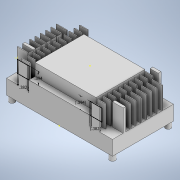
# Autodesk Inventor part: TX2 shape
Saved by Autodesk Inventor 2020 (Build 240168000, 168)
## iProperties
Created: 2019-07-20
Part Number: TX2 shape
Material: Generic
Document SubType Name: Modeling
Designer: Paul
Density: 1 g/cm^3
Appearance: Default
Author: Paul
Autodesk Inventor part; units mm, degrees
ref_plane "YZ Plane" through (0, 0, 0) normal (1, 0, 0) x (0, 1, 0)
ref_plane "XZ Plane" through (0, 0, 0) normal (0, 1, 0) x (-1, 0, 0)
ref_plane "XY Plane" through (0, 0, 0) normal (0, 0, 1) x (1, 0, 0)
sketch "Sketch1" plane through (0, 0, 0) normal (0, 1, 0) x (-1, 0, 0)
  line L0 (43.6, 25.1) -> (-43.6, 25.1)
  line L1 (-43.6, 25.1) -> (-43.6, -25.1)
  line L2 (-43.6, -25.1) -> (43.6, -25.1)
  line L3 (43.6, -25.1) -> (43.6, 25.1)
  line L4 (43.6, 25.1) -> (-43.6, -25.1) construction
  line L5 (-43.6, 25.1) -> (43.6, -25.1) construction
  point P0 (0, 0)
  dimension "d0" = 87.2
  dimension "d1" = 50.2
  constraints: 12 end point, 2 midpoint, 2 parallel, 1 horizontal, 1 perpendicular
  measures "d0" distance of L2.end L1.end
  measures "d1" distance of L1.end L0.end
extrude "Extrusion1" add sketch "Sketch1" along normal blind 30
sketch "Sketch2" plane through (0, 0, 0) normal (0, -1, 0) x (1, 0, 0)
  circle A0 centre (41.3939, 22.8369) radius 2.2
  circle A1 centre (41.3939, -22.8184) radius 2.2
  circle A2 centre (-41.2153, 22.8369) radius 2.2
  circle A3 centre (-41.2153, -22.8184) radius 2.2
  point P0 (0, 0)
  dimension "d4" = 4.4
  dimension "d5" = 4.4
  dimension "d6" = 4.4
  dimension "d7" = 4.4
  constraints: 4 centre point
  measures "d4" diameter of A0
  measures "d5" diameter of A1
  measures "d6" diameter of A2
  measures "d7" diameter of A3
extrude "Extrusion2" add sketch "Sketch2" along normal blind 4.3
sketch "Sketch3" plane through (-43.6, 0, 25.1) normal (0, 0, 1) x (1, 0, 0)
  point P0 (43.6, 0)
sketch "Sketch4" plane through (0, 30, 0) normal (0, 1, 0) x (1, 0, 0)
  line L0 (43.6, 25.1) -> (-43.6, 25.1) projected
  line L1 (43.6, 25.1) -> (34.8, 25.1)
  line L2 (34.8, 25.1) -> (34.8, 16.3)
  line L3 (34.8, 16.3) -> (43.6, 16.3)
  line L4 (43.6, 16.3) -> (43.6, 25.1)
  line L5 (-43.6, 25.1) -> (-34.8, 25.1)
  line L6 (-34.8, 25.1) -> (-34.8, 16.3)
  line L7 (-34.8, 16.3) -> (-43.6, 16.3)
  line L8 (-43.6, 16.3) -> (-43.6, 25.1)
  point P0 (0, 0)
  dimension "d10" = 8.8
  dimension "d11" = 8.8
  dimension "d14" = 8.8
  dimension "d15" = 8.8
  constraints: 16 end point, 4 parallel, 2 horizontal, 2 perpendicular
  measures "d10" distance of L3.end L2.end
  measures "d11" distance of L2.end L1.end
  measures "d14" distance of L6.end L7.end
  measures "d15" distance of L5.end L6.end
sketch "Sketch5" plane through (0, 30, 0) normal (0, 1, 0) x (1, 0, 0)
  line L0 (-43.6, -25.1) -> (43.6, -25.1) projected
  line L1 (43.6, -25.1) -> (34.8, -25.1)
  line L2 (34.8, -25.1) -> (34.8, -16.3)
  line L3 (34.8, -16.3) -> (43.6, -16.3)
  line L4 (43.6, -16.3) -> (43.6, -25.1)
  line L5 (-43.6, 25.1) -> (-43.6, -25.1) projected
  line L6 (-43.6, -25.1) -> (-34.8, -25.1)
  line L7 (-34.8, -25.1) -> (-34.8, -16.3)
  line L8 (-34.8, -16.3) -> (-43.6, -16.3)
  line L9 (-43.6, -16.3) -> (-43.6, -25.1)
  point P0 (0, 0)
  dimension "d18" = 8.8
  dimension "d19" = 8.8
  dimension "d20" = 8.8
  dimension "d21" = 8.8
  constraints: 16 end point, 4 parallel, 2 horizontal, 2 perpendicular
  measures "d18" distance of L2.end L3.end
  measures "d19" distance of L1.end L2.end
  measures "d20" distance of L8.end L7.end
  measures "d21" distance of L7.end L6.end
extrude "Extrusion3" cut sketch "Sketch4" against normal blind 18
extrude "Extrusion4" cut sketch "Sketch5" against normal blind 18
sketch "Sketch6" plane through (43.6, 0, -25.1) normal (0, 0, -1) x (-1, 0, 0)
  line L0 (78.4, 30) -> (8.8, 30) projected
  line L1 (8.8, 30) -> (18.5, 30)
  line L2 (18.5, 30) -> (18.5, 20)
  line L3 (18.5, 20) -> (8.8, 20)
  line L4 (8.8, 20) -> (8.8, 30)
  line L5 (78.4, 30) -> (68.7, 30)
  line L6 (68.7, 30) -> (68.7, 20)
  line L7 (68.7, 20) -> (78.4, 20)
  line L8 (78.4, 20) -> (78.4, 30)
  line L9 (18.5, 30) -> (68.7, 30)
  line L10 (68.7, 30) -> (68.7, 20)
  line L11 (68.7, 20) -> (18.5, 20)
  line L12 (18.5, 20) -> (18.5, 30)
  point P0 (43.6, 0)
  point P1 (18.5, 20)
  point P2 (18.5, 30)
  dimension "d26" = 9.7
  dimension "d27" = 10
  dimension "d28" = 9.7
  dimension "d29" = 10
  constraints: 24 end point, 6 parallel, 3 horizontal, 3 perpendicular
  measures "d26" distance of L2.end L3.end
  measures "d27" distance of L1.end L2.end
  measures "d28" distance of L7.end L6.end
  measures "d29" distance of L6.end L5.end
extrude "Extrusion5" cut sketch "Sketch6" against normal blind 5 contours L6 L11 L2 L0
sketch "Sketch7" plane through (-43.6, 0, 25.1) normal (0, 0, 1) x (1, 0, 0)
  line L0 (0, 30) -> (8.8, 30) projected
  line L1 (8.8, 30) -> (18.5, 30)
  line L2 (18.5, 30) -> (18.5, 20)
  line L3 (18.5, 20) -> (8.8, 20)
  line L4 (8.8, 20) -> (8.8, 30)
  line L5 (78.4, 12) -> (78.4, 30) projected
  line L6 (78.4, 30) -> (68.7, 30)
  line L7 (68.7, 30) -> (68.7, 20)
  line L8 (68.7, 20) -> (78.4, 20)
  line L9 (78.4, 20) -> (78.4, 30)
  line L10 (18.5, 30) -> (68.7, 30)
  line L11 (68.7, 30) -> (68.7, 20)
  line L12 (68.7, 20) -> (18.5, 20)
  line L13 (18.5, 20) -> (18.5, 30)
  point P0 (43.6, 0)
  point P1 (18.5, 20)
  dimension "d32" = 9.7
  dimension "d33" = 10
  dimension "d34" = 9.7
  dimension "d35" = 10
  constraints: 24 end point, 6 parallel, 3 horizontal, 3 perpendicular
  measures "d32" distance of L2.end L3.end
  measures "d33" distance of L1.end L2.end
  measures "d34" distance of L8.end L7.end
  measures "d35" distance of L7.end L6.end
extrude "Extrusion6" cut sketch "Sketch7" along normal blind 5 contours L10 L7 L12 L2
sketch "Sketch8" plane through (-43.6, 0, 25.1) normal (0, 0, 1) x (1, 0, 0)
  point P0 (43.6, 0)
sketch "Sketch9" plane through (-43.6, 0, 25.1) normal (0, 0, 1) x (1, 0, 0)
  line L0 (8.8, 30) -> (18.5, 30)
  line L1 (18.5, 30) -> (18.5, 20)
  line L2 (18.5, 20) -> (8.8, 20)
  line L3 (8.8, 20) -> (8.8, 30)
  line L4 (78.4, 30) -> (68.7, 30) projected
  line L5 (68.7, 20) -> (68.7, 30) projected
  line L6 (78.4, 30) -> (68.7, 30)
  line L7 (68.7, 30) -> (68.7, 20)
  line L8 (68.7, 20) -> (78.4, 20)
  line L9 (78.4, 20) -> (78.4, 30)
  point P0 (43.6, 0)
  dimension "d38" = 9.7
  dimension "d39" = 10
  dimension "d40" = 9.7
  dimension "d41" = 10
  constraints: 16 end point, 4 parallel, 2 horizontal, 2 perpendicular
  measures "d38" distance of L1.end L2.end
  measures "d39" distance of L0.end L1.end
  measures "d40" distance of L8.end L5.start
  measures "d41" distance of L5.start L6.end
sketch "Sketch10" plane through (-43.6, 0, 25.1) normal (0, 0, 1) x (1, 0, 0)
  line L0 (68.7, 30) -> (18.5, 30) projected
  line L1 (18.5, 20) -> (68.7, 20) projected
  line L2 (18.5, 30) -> (68.7, 30)
  line L3 (68.7, 30) -> (68.7, 20)
  line L4 (68.7, 20) -> (18.5, 20)
  line L5 (18.5, 20) -> (18.5, 30)
  point P0 (43.6, 0)
  constraints: 8 end point, 2 parallel, 1 horizontal, 1 perpendicular
extrude "Extrusion7" cut sketch "Sketch10" against normal blind 5
sketch "Sketch11" plane through (0, 30, 0) normal (0, 1, 0) x (1, 0, 0)
  line L0 (25.1, -25.1) -> (-25.1, -25.1) projected
  line L1 (25.1, -25.1) -> (26.6, -25.1)
  line L2 (26.6, -25.1) -> (26.6, 25.1)
  line L3 (26.6, 25.1) -> (25.1, 25.1)
  line L4 (25.1, 25.1) -> (25.1, -25.1)
  line L5 (-25.1, -25.1) -> (-26.6, -25.1)
  line L6 (-26.6, -25.1) -> (-26.6, 25.1)
  line L7 (-26.6, 25.1) -> (-25.1, 25.1)
  line L8 (-25.1, 25.1) -> (-25.1, -25.1)
  point P0 (0, 0)
  dimension "d44" = 1.5
  dimension "d45" = 50.2
  dimension "d46" = 1.5
  constraints: 16 end point, 4 parallel, 2 horizontal, 2 perpendicular
  measures "d44" distance of L3.end L2.end
  measures "d45" distance of L2.end L1.end
  measures "d46" distance of L6.end L7.end
extrude "Extrusion8" cut sketch "Sketch11" against normal blind 18
sketch "Sketch12" plane through (0, 30, 0) normal (0, 1, 0) x (1, 0, 0)
  line L0 (-34.8, 25.1) -> (-33.3, 25.1)
  line L1 (-33.3, 25.1) -> (-33.3, -25.1)
  line L2 (-33.3, -25.1) -> (-34.8, -25.1)
  line L3 (-34.8, -25.1) -> (-34.8, 25.1)
  line L4 (34.8, 25.1) -> (43.6, 25.1) projected
  line L5 (34.8, 25.1) -> (33.3, 25.1)
  line L6 (33.3, 25.1) -> (33.3, -25.1)
  line L7 (33.3, -25.1) -> (34.8, -25.1)
  line L8 (34.8, -25.1) -> (34.8, 25.1)
  point P0 (0, 0)
  dimension "d50" = 1.5
  dimension "d51" = 50.2
  dimension "d52" = 1.5
  dimension "d53" = 50.2
  constraints: 16 end point, 4 parallel, 2 horizontal, 2 perpendicular
  measures "d50" distance of L1.end L2.end
  measures "d51" distance of L0.end L1.end
  measures "d52" distance of L7.end L6.end
  measures "d53" distance of L6.end L5.end
extrude "Extrusion9" cut sketch "Sketch12" against normal blind 18
sketch "Sketch13" plane through (0, 30, 0) normal (0, 1, 0) x (1, 0, 0)
  line L0 (-34.8, -16.3) -> (-34.8, 16.3) projected
  line L1 (-43.6, 16.3) -> (-43.6, -16.3) projected
  line L2 (-43.6, 16.3) -> (-34.81, 16.3)
  line L3 (-34.81, 16.3) -> (-34.81, 15.65)
  line L4 (-34.81, 15.65) -> (-43.6, 15.65)
  line L5 (-43.6, 15.65) -> (-43.6, 16.3)
  line L6 (-43.6, 15.65) -> (179.412, 15.65)
  line L7 (179.412, 15.65) -> (179.412, 11.95)
  line L8 (179.412, 11.95) -> (-43.6, 11.95)
  line L9 (-43.6, 11.95) -> (-43.6, 15.65)
  line L10 (-43.6, 11.95) -> (-34.81, 11.95)
  line L11 (-34.81, 11.95) -> (-34.81, 11.3)
  line L12 (-34.81, 11.3) -> (-43.6, 11.3)
  line L13 (-43.6, 11.3) -> (-43.6, 11.95)
  line L14 (-43.6, 11.3) -> (-34.81, 11.3)
  line L15 (-34.81, 11.3) -> (-34.81, 7.6)
  line L16 (-34.81, 7.6) -> (-43.6, 7.6)
  line L17 (-43.6, 7.6) -> (-43.6, 11.3)
  line L18 (-43.6, 7.6) -> (-34.81, 7.6)
  line L19 (-34.81, 7.6) -> (-34.81, 6.95)
  line L20 (-34.81, 6.95) -> (-43.6, 6.95)
  line L21 (-43.6, 6.95) -> (-43.6, 7.6)
  line L22 (-43.6, 6.95) -> (-34.81, 6.95)
  line L23 (-34.81, 6.95) -> (-34.81, 3.25)
  line L24 (-34.81, 3.25) -> (-43.6, 3.25)
  line L25 (-43.6, 3.25) -> (-43.6, 6.95)
  line L26 (-43.6, 3.25) -> (-34.81, 3.25)
  line L27 (-34.81, 3.25) -> (-34.81, 2.6)
  line L28 (-34.81, 2.6) -> (-43.6, 2.6)
  line L29 (-43.6, 2.6) -> (-43.6, 3.25)
  line L30 (-43.6, 2.6) -> (-34.81, 2.6)
  line L31 (-34.81, 2.6) -> (-34.81, -1.1)
  line L32 (-34.81, -1.1) -> (-43.6, -1.1)
  line L33 (-43.6, -1.1) -> (-43.6, 2.6)
  line L34 (-43.6, -1.1) -> (-34.81, -1.1)
  line L35 (-34.81, -1.1) -> (-34.81, -1.75)
  line L36 (-34.81, -1.75) -> (-43.6, -1.75)
  line L37 (-43.6, -1.75) -> (-43.6, -1.1)
  line L38 (-43.6, -1.75) -> (-34.81, -1.75)
  line L39 (-34.81, -1.75) -> (-34.81, -5.45)
  line L40 (-34.81, -5.45) -> (-43.6, -5.45)
  line L41 (-43.6, -5.45) -> (-43.6, -1.75)
  line L42 (-43.6, -5.45) -> (-34.81, -5.45)
  line L43 (-34.81, -5.45) -> (-34.81, -6.1)
  line L44 (-34.81, -6.1) -> (-43.6, -6.1)
  line L45 (-43.6, -6.1) -> (-43.6, -5.45)
  line L46 (-43.6, -6.1) -> (-34.81, -6.1)
  line L47 (-34.81, -6.1) -> (-34.81, -9.8)
  line L48 (-34.81, -9.8) -> (-43.6, -9.8)
  line L49 (-43.6, -9.8) -> (-43.6, -6.1)
  line L50 (-43.6, -9.8) -> (-34.81, -9.8)
  line L51 (-34.81, -9.8) -> (-34.81, -10.45)
  line L52 (-34.81, -10.45) -> (-43.6, -10.45)
  line L53 (-43.6, -10.45) -> (-43.6, -9.8)
  line L54 (-43.6, -16.3) -> (-34.8, -16.3) projected
  line L55 (-43.6, -16.3) -> (-34.81, -16.3)
  line L56 (-34.81, -16.3) -> (-34.81, -15.65)
  line L57 (-34.81, -15.65) -> (-43.6, -15.65)
  line L58 (-43.6, -15.65) -> (-43.6, -16.3)
  line L59 (-43.6, -15.65) -> (-34.81, -15.65)
  line L60 (-34.81, -15.65) -> (-34.81, -11.95)
  line L61 (-34.81, -11.95) -> (-43.6, -11.95)
  line L62 (-43.6, -11.95) -> (-43.6, -15.65)
  point P0 (0, 0)
  point P1 (-34.8, 11.95)
  point P2 (-34.8, 15.65)
  point P3 (-43.6, 11.95)
  dimension "d56" = 8.8
  dimension "d57" = 8.79
  dimension "d58" = 0.65
  dimension "d59" = 223.012
  dimension "d60" = 3.7
  dimension "d61" = 8.79
  dimension "d62" = 0.65
  dimension "d63" = 8.79
  dimension "d64" = 3.7
  dimension "d65" = 8.79
  dimension "d66" = 0.65
  dimension "d67" = 8.79
  dimension "d68" = 3.7
  dimension "d69" = 8.79
  dimension "d70" = 0.65
  dimension "d71" = 8.79
  dimension "d72" = 3.7
  dimension "d73" = 8.79
  dimension "d74" = 0.65
  dimension "d75" = 8.79
  dimension "d76" = 3.7
  dimension "d77" = 8.79
  dimension "d78" = 0.65
  dimension "d79" = 8.79
  dimension "d80" = 3.7
  dimension "d81" = 8.79
  dimension "d82" = 0.65
  dimension "d83" = 8.79
  dimension "d84" = 0.65
  dimension "d85" = 8.79
  dimension "d86" = 3.7
  constraints: 120 end point, 30 parallel, 15 horizontal, 15 perpendicular
  measures "d56" distance between parallel lines of L0 L1
  measures "d57" distance of L3.end L4.end
  measures "d58" distance of L2.end L3.end
  measures "d59" distance of L7.end L8.end
  measures "d60" distance of L6.end L7.end
  measures "d61" distance of L11.end L12.end
  measures "d62" distance of L10.end L11.end
  measures "d63" distance of L15.end L16.end
  measures "d64" distance of L14.end L15.end
  measures "d65" distance of L19.end L20.end
  measures "d66" distance of L18.end L19.end
  measures "d67" distance of L23.end L24.end
  measures "d68" distance of L22.end L23.end
  measures "d69" distance of L27.end L28.end
  measures "d70" distance of L26.end L27.end
  measures "d71" distance of L31.end L32.end
  measures "d72" distance of L30.end L31.end
  measures "d73" distance of L35.end L36.end
  measures "d74" distance of L34.end L35.end
  measures "d75" distance of L39.end L40.end
  measures "d76" distance of L38.end L39.end
  measures "d77" distance of L43.end L44.end
  measures "d78" distance of L42.end L43.end
  measures "d79" distance of L47.end L48.end
  measures "d80" distance of L46.end L47.end
  measures "d81" distance of L51.end L52.end
  measures "d82" distance of L50.end L51.end
  measures "d83" distance of L57.end L56.end
  measures "d84" distance of L56.end L55.end
  measures "d85" distance of L61.end L60.end
  measures "d86" distance of L60.end L59.end
extrude "Extrusion10" cut sketch "Sketch13" against normal blind 18 contours L8 L1 L4 L6 L0 | L57 L1 L61 L60 | L15 L16 L1 L12 | L23 L24 L1 L20 | L1 L44 L47 L48 | L31 L32 L1 L28 | L1 L36 L39 L40
sketch "Sketch14" plane through (0, 30, 0) normal (0, 1, 0) x (1, 0, 0)
  line L0 (43.6, 16.3) -> (34.8, 16.3) projected
  line L1 (34.8, 16.3) -> (43.6, 16.3)
  line L2 (43.6, 16.3) -> (43.6, 15.65)
  line L3 (43.6, 15.65) -> (34.8, 15.65)
  line L4 (34.8, 15.65) -> (34.8, 16.3)
  line L5 (34.8, 15.65) -> (43.6, 15.65)
  line L6 (43.6, 15.65) -> (43.6, 11.95)
  line L7 (43.6, 11.95) -> (34.8, 11.95)
  line L8 (34.8, 11.95) -> (34.8, 15.65)
  line L9 (34.8, 11.95) -> (43.6, 11.95)
  line L10 (43.6, 11.95) -> (43.6, 11.3)
  line L11 (43.6, 11.3) -> (34.8, 11.3)
  line L12 (34.8, 11.3) -> (34.8, 11.95)
  point P0 (0, 0)
  dimension "d89" = 8.8
  dimension "d90" = 0.65
  dimension "d91" = 8.8
  dimension "d92" = 3.7
  dimension "d93" = 8.8
  dimension "d94" = 0.65
  constraints: 24 end point, 6 parallel, 3 horizontal, 3 perpendicular
  measures "d89" distance of L2.end L3.end
  measures "d90" distance of L1.end L2.end
  measures "d91" distance of L6.end L7.end
  measures "d92" distance of L5.end L6.end
  measures "d93" distance of L10.end L11.end
  measures "d94" distance of L9.end L10.end
extrude "Extrusion11" cut sketch "Sketch14" against normal blind 18 contours L6 L7 L8 L3
sketch "Sketch15" plane through (0, 30, 0) normal (0, 1, 0) x (1, 0, 0)
  line L0 (43.6, 11.95) -> (34.8, 11.95) projected
  line L1 (34.8, 11.95) -> (43.6, 11.95)
  line L2 (43.6, 11.95) -> (43.6, 11.3)
  line L3 (43.6, 11.3) -> (34.8, 11.3)
  line L4 (34.8, 11.3) -> (34.8, 11.95)
  line L5 (34.8, 11.3) -> (43.6, 11.3)
  line L6 (43.6, 11.3) -> (43.6, 7.6)
  line L7 (43.6, 7.6) -> (34.8, 7.6)
  line L8 (34.8, 7.6) -> (34.8, 11.3)
  line L9 (34.8, 7.6) -> (43.6, 7.6)
  line L10 (43.6, 7.6) -> (43.6, 6.95)
  line L11 (43.6, 6.95) -> (34.8, 6.95)
  line L12 (34.8, 6.95) -> (34.8, 7.6)
  line L13 (34.8, 6.95) -> (43.6, 6.95)
  line L14 (43.6, 6.95) -> (43.6, 3.25)
  line L15 (43.6, 3.25) -> (34.8, 3.25)
  line L16 (34.8, 3.25) -> (34.8, 6.95)
  line L17 (34.8, 3.25) -> (43.6, 3.25)
  line L18 (43.6, 3.25) -> (43.6, 2.6)
  line L19 (43.6, 2.6) -> (34.8, 2.6)
  line L20 (34.8, 2.6) -> (34.8, 3.25)
  line L21 (34.8, 2.6) -> (43.6, 2.6)
  line L22 (43.6, 2.6) -> (43.6, -1.1)
  line L23 (43.6, -1.1) -> (34.8, -1.1)
  line L24 (34.8, -1.1) -> (34.8, 2.6)
  line L25 (34.8, -1.1) -> (43.6, -1.1)
  line L26 (43.6, -1.1) -> (43.6, -1.75)
  line L27 (43.6, -1.75) -> (34.8, -1.75)
  line L28 (34.8, -1.75) -> (34.8, -1.1)
  line L29 (34.8, -1.75) -> (43.6, -1.75)
  line L30 (43.6, -1.75) -> (43.6, -5.45)
  line L31 (43.6, -5.45) -> (34.8, -5.45)
  line L32 (34.8, -5.45) -> (34.8, -1.75)
  line L33 (34.8, -5.45) -> (43.6, -5.45)
  line L34 (43.6, -5.45) -> (43.6, -6.1)
  line L35 (43.6, -6.1) -> (34.8, -6.1)
  line L36 (34.8, -6.1) -> (34.8, -5.45)
  line L37 (34.8, -6.1) -> (43.6, -6.1)
  line L38 (43.6, -6.1) -> (43.6, -9.8)
  line L39 (43.6, -9.8) -> (34.8, -9.8)
  line L40 (34.8, -9.8) -> (34.8, -6.1)
  line L41 (34.8, -9.8) -> (43.6, -9.8)
  line L42 (43.6, -9.8) -> (43.6, -10.45)
  line L43 (43.6, -10.45) -> (34.8, -10.45)
  line L44 (34.8, -10.45) -> (34.8, -9.8)
  line L45 (34.8, 11.95) -> (34.8, -16.3) projected
  line L46 (34.8, -16.3) -> (43.6, -16.3)
  line L47 (43.6, -16.3) -> (43.6, -15.65)
  line L48 (43.6, -15.65) -> (34.8, -15.65)
  line L49 (34.8, -15.65) -> (34.8, -16.3)
  line L50 (34.8, -10.45) -> (43.6, -10.45)
  line L51 (43.6, -10.45) -> (43.6, -14.15)
  line L52 (43.6, -14.15) -> (34.8, -14.15)
  line L53 (34.8, -14.15) -> (34.8, -10.45)
  point P0 (0, 0)
  dimension "d97" = 8.8
  dimension "d98" = 0.65
  dimension "d99" = 8.8
  dimension "d100" = 3.7
  dimension "d101" = 8.8
  dimension "d102" = 0.65
  dimension "d103" = 8.8
  dimension "d104" = 3.7
  dimension "d105" = 8.8
  dimension "d106" = 0.65
  dimension "d107" = 8.8
  dimension "d108" = 3.7
  dimension "d109" = 8.8
  dimension "d110" = 0.65
  dimension "d111" = 8.8
  dimension "d112" = 3.7
  dimension "d113" = 8.8
  dimension "d114" = 0.65
  dimension "d115" = 8.8
  dimension "d116" = 3.7
  dimension "d117" = 8.8
  dimension "d118" = 0.65
  dimension "d119" = 8.8
  dimension "d120" = 0.65
  dimension "d121" = 8.8
  dimension "d122" = 3.7
  constraints: 104 end point, 26 parallel, 13 horizontal, 13 perpendicular, 1 other
  measures "d97" distance of L2.end L3.end
  measures "d98" distance of L1.end L2.end
  measures "d99" distance of L6.end L7.end
  measures "d100" distance of L5.end L6.end
  measures "d101" distance of L10.end L11.end
  measures "d102" distance of L9.end L10.end
  measures "d103" distance of L14.end L15.end
  measures "d104" distance of L13.end L14.end
  measures "d105" distance of L18.end L19.end
  measures "d106" distance of L17.end L18.end
  measures "d107" distance of L22.end L23.end
  measures "d108" distance of L21.end L22.end
  measures "d109" distance of L26.end L27.end
  measures "d110" distance of L25.end L26.end
  measures "d111" distance of L30.end L31.end
  measures "d112" distance of L29.end L30.end
  measures "d113" distance of L34.end L35.end
  measures "d114" distance of L33.end L34.end
  measures "d115" distance of L38.end L39.end
  measures "d116" distance of L37.end L38.end
  measures "d117" distance of L42.end L43.end
  measures "d118" distance of L41.end L42.end
  measures "d119" distance of L48.end L47.end
  measures "d120" distance of L47.end L46.end
  measures "d121" distance of L51.end L52.end
  measures "d122" distance of L50.end L51.end
extrude "Extrusion12" cut sketch "Sketch15" against normal blind 18 contours L6 L7 L8 L3 | L14 L15 L16 L11 | L22 L23 L24 L19 | L30 L31 L32 L27 | L38 L39 L40 L35 | L51 L52 L45 L43
sketch "Sketch16" plane through (0, 30, 0) normal (0, 1, 0) x (1, 0, 0)
  line L0 (-33.3, 25.1) -> (-33.3, -25.1) projected
  line L1 (-26.6, -25.1) -> (-26.6, 25.1) projected
  line L2 (-33.3, 25.1) -> (-26.59, 25.1)
  line L3 (-26.59, 25.1) -> (-26.59, 24.45)
  line L4 (-26.59, 24.45) -> (-33.3, 24.45)
  line L5 (-33.3, 24.45) -> (-33.3, 25.1)
  line L6 (-33.3, 24.45) -> (-26.59, 24.45)
  line L7 (-26.59, 24.45) -> (-26.59, 20.75)
  line L8 (-26.59, 20.75) -> (-33.3, 20.75)
  line L9 (-33.3, 20.75) -> (-33.3, 24.45)
  line L10 (-33.3, 20.75) -> (-26.59, 20.75)
  line L11 (-26.59, 20.75) -> (-26.59, 20.1)
  line L12 (-26.59, 20.1) -> (-33.3, 20.1)
  line L13 (-33.3, 20.1) -> (-33.3, 20.75)
  point P0 (0, 0)
  point P1 (-26.6, 20.75)
  point P2 (-26.6, 24.45)
  dimension "d125" = 6.71
  dimension "d126" = 0.65
  dimension "d127" = 6.71
  dimension "d128" = 3.7
  dimension "d129" = 6.71
  dimension "d130" = 0.65
  constraints: 24 end point, 6 parallel, 3 horizontal, 3 perpendicular
  measures "d125" distance of L3.end L4.end
  measures "d126" distance of L2.end L3.end
  measures "d127" distance of L7.end L8.end
  measures "d128" distance of L6.end L7.end
  measures "d129" distance of L11.end L12.end
  measures "d130" distance of L10.end L11.end
extrude "Extrusion13" cut sketch "Sketch16" against normal blind 18 contours L4 L1 L8 L0
sketch "Sketch17" plane through (0, 30, 0) normal (0, 1, 0) x (1, 0, 0)
  line L0 (-26.6, 20.75) -> (-33.3, 20.75) projected
  line L1 (-33.3, 20.75) -> (-26.59, 20.75)
  line L2 (-26.59, 20.75) -> (-26.59, 20.1)
  line L3 (-26.59, 20.1) -> (-33.3, 20.1)
  line L4 (-33.3, 20.1) -> (-33.3, 20.75)
  line L5 (-33.3, 20.1) -> (-26.59, 20.1)
  line L6 (-26.59, 20.1) -> (-26.59, 16.4)
  line L7 (-26.59, 16.4) -> (-33.3, 16.4)
  line L8 (-33.3, 16.4) -> (-33.3, 20.1)
  line L9 (-33.3, 16.4) -> (-26.59, 16.4)
  line L10 (-26.59, 16.4) -> (-26.59, 15.75)
  line L11 (-26.59, 15.75) -> (-33.3, 15.75)
  line L12 (-33.3, 15.75) -> (-33.3, 16.4)
  line L13 (-33.3, 15.75) -> (-26.59, 15.75)
  line L14 (-26.59, 15.75) -> (-26.59, 12.05)
  line L15 (-26.59, 12.05) -> (-33.3, 12.05)
  line L16 (-33.3, 12.05) -> (-33.3, 15.75)
  line L17 (-33.3, 12.05) -> (-26.59, 12.05)
  line L18 (-26.59, 12.05) -> (-26.59, 11.4)
  line L19 (-26.59, 11.4) -> (-33.3, 11.4)
  line L20 (-33.3, 11.4) -> (-33.3, 12.05)
  line L21 (-33.3, 11.4) -> (-26.59, 11.4)
  line L22 (-26.59, 11.4) -> (-26.59, 7.7)
  line L23 (-26.59, 7.7) -> (-33.3, 7.7)
  line L24 (-33.3, 7.7) -> (-33.3, 11.4)
  line L25 (-33.3, 7.7) -> (-26.59, 7.7)
  line L26 (-26.59, 7.7) -> (-26.59, 7.05)
  line L27 (-26.59, 7.05) -> (-33.3, 7.05)
  line L28 (-33.3, 7.05) -> (-33.3, 7.7)
  line L29 (-33.3, 7.05) -> (-26.59, 7.05)
  line L30 (-26.59, 7.05) -> (-26.59, 3.35)
  line L31 (-26.59, 3.35) -> (-33.3, 3.35)
  line L32 (-33.3, 3.35) -> (-33.3, 7.05)
  line L33 (-33.3, 3.35) -> (-26.59, 3.35)
  line L34 (-26.59, 3.35) -> (-26.59, 2.7)
  line L35 (-26.59, 2.7) -> (-33.3, 2.7)
  line L36 (-33.3, 2.7) -> (-33.3, 3.35)
  line L37 (-33.3, 2.7) -> (-26.59, 2.7)
  line L38 (-26.59, 2.7) -> (-26.59, -1)
  line L39 (-26.59, -1) -> (-33.3, -1)
  line L40 (-33.3, -1) -> (-33.3, 2.7)
  line L41 (-33.3, -1) -> (-26.59, -1)
  line L42 (-26.59, -1) -> (-26.59, -1.65)
  line L43 (-26.59, -1.65) -> (-33.3, -1.65)
  line L44 (-33.3, -1.65) -> (-33.3, -1)
  line L45 (-33.3, -1.65) -> (-26.59, -1.65)
  line L46 (-26.59, -1.65) -> (-26.59, -5.35)
  line L47 (-26.59, -5.35) -> (-33.3, -5.35)
  line L48 (-33.3, -5.35) -> (-33.3, -1.65)
  line L49 (-33.3, -5.35) -> (-26.59, -5.35)
  line L50 (-26.59, -5.35) -> (-26.59, -6)
  line L51 (-26.59, -6) -> (-33.3, -6)
  line L52 (-33.3, -6) -> (-33.3, -5.35)
  line L53 (-33.3, -6) -> (-26.59, -6)
  line L54 (-26.59, -6) -> (-26.59, -9.7)
  line L55 (-26.59, -9.7) -> (-33.3, -9.7)
  line L56 (-33.3, -9.7) -> (-33.3, -6)
  line L57 (-33.3, -9.7) -> (-26.59, -9.7)
  line L58 (-26.59, -9.7) -> (-26.59, -10.35)
  line L59 (-26.59, -10.35) -> (-33.3, -10.35)
  line L60 (-33.3, -10.35) -> (-33.3, -9.7)
  line L61 (-33.3, -10.35) -> (-26.59, -10.35)
  line L62 (-26.59, -10.35) -> (-26.59, -13.4782)
  line L63 (-26.59, -13.4782) -> (-33.3, -13.4782)
  line L64 (-33.3, -13.4782) -> (-33.3, -10.35)
  line L65 (-33.3, -13.4782) -> (-26.59, -13.4782)
  line L66 (-26.59, -13.4782) -> (-26.59, -14.1282)
  line L67 (-26.59, -14.1282) -> (-33.3, -14.1282)
  line L68 (-33.3, -14.1282) -> (-33.3, -13.4782)
  line L69 (-33.3, -14.1282) -> (-26.59, -14.1282)
  line L70 (-26.59, -14.1282) -> (-26.59, -17.8282)
  line L71 (-26.59, -17.8282) -> (-33.3, -17.8282)
  line L72 (-33.3, -17.8282) -> (-33.3, -14.1282)
  line L73 (-33.3, -17.8282) -> (-26.59, -17.8282)
  line L74 (-26.59, -17.8282) -> (-26.59, -18.4782)
  line L75 (-26.59, -18.4782) -> (-33.3, -18.4782)
  line L76 (-33.3, -18.4782) -> (-33.3, -17.8282)
  line L77 (-33.3, -18.4782) -> (-26.59, -18.4782)
  line L78 (-26.59, -18.4782) -> (-26.59, -22.1782)
  line L79 (-26.59, -22.1782) -> (-33.3, -22.1782)
  line L80 (-33.3, -22.1782) -> (-33.3, -18.4782)
  line L81 (-33.3, -22.1782) -> (-26.59, -22.1782)
  line L82 (-26.59, -22.1782) -> (-26.59, -22.8282)
  line L83 (-26.59, -22.8282) -> (-33.3, -22.8282)
  line L84 (-33.3, -22.8282) -> (-33.3, -22.1782)
  line L85 (-33.3, 20.75) -> (-33.3, -25.1) projected
  line L86 (-33.3, -25.1) -> (-26.59, -25.1)
  line L87 (-26.59, -25.1) -> (-26.59, -24.45)
  line L88 (-26.59, -24.45) -> (-33.3, -24.45)
  line L89 (-33.3, -24.45) -> (-33.3, -25.1)
  point P0 (0, 0)
  dimension "d133" = 6.71
  dimension "d134" = 0.65
  dimension "d135" = 6.71
  dimension "d136" = 3.7
  dimension "d137" = 6.71
  dimension "d138" = 0.65
  dimension "d139" = 6.71
  dimension "d140" = 3.7
  dimension "d141" = 6.71
  dimension "d142" = 0.65
  dimension "d143" = 6.71
  dimension "d144" = 3.7
  dimension "d145" = 6.71
  dimension "d146" = 0.65
  dimension "d147" = 6.71
  dimension "d148" = 3.7
  dimension "d149" = 6.71
  dimension "d150" = 0.65
  dimension "d151" = 6.71
  dimension "d152" = 3.7
  dimension "d153" = 6.71
  dimension "d154" = 0.65
  dimension "d155" = 6.71
  dimension "d156" = 3.7
  dimension "d157" = 6.71
  dimension "d158" = 0.65
  dimension "d159" = 6.71
  dimension "d160" = 3.7
  dimension "d161" = 6.71
  dimension "d162" = 0.65
  dimension "d163" = 6.71
  dimension "d164" = 6.71
  dimension "d165" = 0.65
  dimension "d166" = 6.71
  dimension "d167" = 3.7
  dimension "d168" = 6.71
  dimension "d169" = 0.65
  dimension "d170" = 6.71
  dimension "d171" = 3.7
  dimension "d172" = 6.71
  dimension "d173" = 0.65
  dimension "d174" = 6.71
  dimension "d175" = 0.65
  constraints: 176 end point, 44 parallel, 22 horizontal, 22 perpendicular, 1 other
  measures "d133" distance of L2.end L3.end
  measures "d134" distance of L1.end L2.end
  measures "d135" distance of L6.end L7.end
  measures "d136" distance of L5.end L6.end
  measures "d137" distance of L10.end L11.end
  measures "d138" distance of L9.end L10.end
  measures "d139" distance of L14.end L15.end
  measures "d140" distance of L13.end L14.end
  measures "d141" distance of L18.end L19.end
  measures "d142" distance of L17.end L18.end
  measures "d143" distance of L22.end L23.end
  measures "d144" distance of L21.end L22.end
  measures "d145" distance of L26.end L27.end
  measures "d146" distance of L25.end L26.end
  measures "d147" distance of L30.end L31.end
  measures "d148" distance of L29.end L30.end
  measures "d149" distance of L34.end L35.end
  measures "d150" distance of L33.end L34.end
  measures "d151" distance of L38.end L39.end
  measures "d152" distance of L37.end L38.end
  measures "d153" distance of L42.end L43.end
  measures "d154" distance of L41.end L42.end
  measures "d155" distance of L46.end L47.end
  measures "d156" distance of L45.end L46.end
  measures "d157" distance of L50.end L51.end
  measures "d158" distance of L49.end L50.end
  measures "d159" distance of L54.end L55.end
  measures "d160" distance of L53.end L54.end
  measures "d161" distance of L58.end L59.end
  measures "d162" distance of L57.end L58.end
  measures "d163" distance of L62.end L63.end
  measures "d164" distance of L66.end L67.end
  measures "d165" distance of L65.end L66.end
  measures "d166" distance of L70.end L71.end
  measures "d167" distance of L69.end L70.end
  measures "d168" distance of L74.end L75.end
  measures "d169" distance of L73.end L74.end
  measures "d170" distance of L78.end L79.end
  measures "d171" distance of L77.end L78.end
  measures "d172" distance of L82.end L83.end
  measures "d173" distance of L81.end L82.end
  measures "d174" distance of L88.end L87.end
  measures "d175" distance of L87.end L86.end
extrude "Extrusion14" cut sketch "Sketch17" against normal blind 18 contours L3 L6 L7 L8 | L11 L14 L15 L16 | L19 L22 L23 L24 | L27 L30 L31 L32 | L35 L38 L39 L40 | L43 L46 L47 L48 | L51 L54 L55 L56 | L59 L62 L63 L64 | L67 L70 L71 L72 | L75 L78 L79 L80
sketch "Sketch18" plane through (0, 30, 0) normal (0, 1, 0) x (1, 0, 0)
  line L0 (-33.3, -22.1782) -> (-33.3, -25.1) projected
  line L1 (-33.3, -22.1782) -> (-26.59, -22.1782)
  line L2 (-26.59, -22.1782) -> (-26.59, -22.8282)
  line L3 (-26.59, -22.8282) -> (-33.3, -22.8282)
  line L4 (-33.3, -22.8282) -> (-33.3, -22.1782)
  line L5 (-33.3, -25.1) -> (-43.6, -25.1) projected
  line L6 (-33.3, -25.1) -> (-26.59, -25.1)
  line L7 (-26.59, -25.1) -> (-26.59, -24.45)
  line L8 (-26.59, -24.45) -> (-33.3, -24.45)
  line L9 (-33.3, -24.45) -> (-33.3, -25.1)
  line L10 (-33.3, -22.8282) -> (-26.59, -22.8282)
  line L11 (-26.59, -22.8282) -> (-26.59, -24.45)
  line L12 (-26.59, -24.45) -> (-33.3, -24.45)
  line L13 (-33.3, -24.45) -> (-33.3, -22.8282)
  point P0 (0, 0)
  dimension "d178" = 6.71
  dimension "d179" = 0.65
  dimension "d180" = 6.71
  dimension "d181" = 0.65
  constraints: 24 end point, 6 parallel, 3 horizontal, 3 perpendicular
  measures "d178" distance of L2.end L3.end
  measures "d179" distance of L1.end L2.end
  measures "d180" distance of L8.end L7.end
  measures "d181" distance of L7.end L6.end
extrude "Extrusion15" cut sketch "Sketch18" against normal blind 18 contours L3 L11 L8 L0
sketch "Sketch19" plane through (0, 30, 0) normal (0, 1, 0) x (1, 0, 0)
  line L0 (33.3, -25.1) -> (33.3, 25.1) projected
  line L1 (33.3, -25.1) -> (26.59, -25.1)
  line L2 (26.59, -25.1) -> (26.59, -24.45)
  line L3 (26.59, -24.45) -> (33.3, -24.45)
  line L4 (33.3, -24.45) -> (33.3, -25.1)
  line L5 (33.3, -24.45) -> (26.59, -24.45)
  line L6 (26.59, -24.45) -> (26.59, -20.75)
  line L7 (26.59, -20.75) -> (33.3, -20.75)
  line L8 (33.3, -20.75) -> (33.3, -24.45)
  line L9 (33.3, -20.75) -> (26.59, -20.75)
  line L10 (26.59, -20.75) -> (26.59, -20.1)
  line L11 (26.59, -20.1) -> (33.3, -20.1)
  line L12 (33.3, -20.1) -> (33.3, -20.75)
  line L13 (33.3, -20.1) -> (26.59, -20.1)
  line L14 (26.59, -20.1) -> (26.59, -16.4)
  line L15 (26.59, -16.4) -> (33.3, -16.4)
  line L16 (33.3, -16.4) -> (33.3, -20.1)
  line L17 (33.3, -16.4) -> (26.59, -16.4)
  line L18 (26.59, -16.4) -> (26.59, -15.75)
  line L19 (26.59, -15.75) -> (33.3, -15.75)
  line L20 (33.3, -15.75) -> (33.3, -16.4)
  line L21 (33.3, -15.75) -> (26.59, -15.75)
  line L22 (26.59, -15.75) -> (26.59, -12.05)
  line L23 (26.59, -12.05) -> (33.3, -12.05)
  line L24 (33.3, -12.05) -> (33.3, -15.75)
  line L25 (33.3, -12.05) -> (26.59, -12.05)
  line L26 (26.59, -12.05) -> (26.59, -11.4)
  line L27 (26.59, -11.4) -> (33.3, -11.4)
  line L28 (33.3, -11.4) -> (33.3, -12.05)
  line L29 (33.3, -11.4) -> (26.59, -11.4)
  line L30 (26.59, -11.4) -> (26.59, -7.7)
  line L31 (26.59, -7.7) -> (33.3, -7.7)
  line L32 (33.3, -7.7) -> (33.3, -11.4)
  line L33 (33.3, -7.7) -> (26.59, -7.7)
  line L34 (26.59, -7.7) -> (26.59, -7.05)
  line L35 (26.59, -7.05) -> (33.3, -7.05)
  line L36 (33.3, -7.05) -> (33.3, -7.7)
  line L37 (33.3, -7.05) -> (26.59, -7.05)
  line L38 (26.59, -7.05) -> (26.59, -3.35)
  line L39 (26.59, -3.35) -> (33.3, -3.35)
  line L40 (33.3, -3.35) -> (33.3, -7.05)
  line L41 (33.3, -3.35) -> (26.59, -3.35)
  line L42 (26.59, -3.35) -> (26.59, -2.7)
  line L43 (26.59, -2.7) -> (33.3, -2.7)
  line L44 (33.3, -2.7) -> (33.3, -3.35)
  line L45 (33.3, -2.7) -> (26.59, -2.7)
  line L46 (26.59, -2.7) -> (26.59, 1)
  line L47 (26.59, 1) -> (33.3, 1)
  line L48 (33.3, 1) -> (33.3, -2.7)
  line L49 (33.3, 1) -> (26.59, 1)
  line L50 (26.59, 1) -> (26.59, 1.65)
  line L51 (26.59, 1.65) -> (33.3, 1.65)
  line L52 (33.3, 1.65) -> (33.3, 1)
  line L53 (33.3, 1.65) -> (26.59, 1.65)
  line L54 (26.59, 1.65) -> (26.59, 5.35)
  line L55 (26.59, 5.35) -> (33.3, 5.35)
  line L56 (33.3, 5.35) -> (33.3, 1.65)
  line L57 (33.3, 5.35) -> (26.59, 5.35)
  line L58 (26.59, 5.35) -> (26.59, 6)
  line L59 (26.59, 6) -> (33.3, 6)
  line L60 (33.3, 6) -> (33.3, 5.35)
  line L61 (33.3, 6) -> (26.59, 6)
  line L62 (26.59, 6) -> (26.59, 9.7)
  line L63 (26.59, 9.7) -> (33.3, 9.7)
  line L64 (33.3, 9.7) -> (33.3, 6)
  line L65 (33.3, 9.7) -> (26.59, 9.7)
  line L66 (26.59, 9.7) -> (26.59, 10.35)
  line L67 (26.59, 10.35) -> (33.3, 10.35)
  line L68 (33.3, 10.35) -> (33.3, 9.7)
  line L69 (33.3, 10.35) -> (26.59, 10.35)
  line L70 (26.59, 10.35) -> (26.59, 14.05)
  line L71 (26.59, 14.05) -> (33.3, 14.05)
  line L72 (33.3, 14.05) -> (33.3, 10.35)
  line L73 (33.3, 14.05) -> (26.59, 14.05)
  line L74 (26.59, 14.05) -> (26.59, 14.7)
  line L75 (26.59, 14.7) -> (33.3, 14.7)
  line L76 (33.3, 14.7) -> (33.3, 14.05)
  line L77 (33.3, 25.1) -> (26.59, 25.1)
  line L78 (26.59, 25.1) -> (26.59, 24.45)
  line L79 (26.59, 24.45) -> (33.3, 24.45)
  line L80 (33.3, 24.45) -> (33.3, 25.1)
  line L81 (33.3, 14.7) -> (26.59, 14.7)
  line L82 (26.59, 14.7) -> (26.59, 18.4)
  line L83 (26.59, 18.4) -> (33.3, 18.4)
  line L84 (33.3, 18.4) -> (33.3, 14.7)
  line L85 (33.3, 18.4) -> (26.59, 18.4)
  line L86 (26.59, 18.4) -> (26.59, 19.05)
  line L87 (26.59, 19.05) -> (33.3, 19.05)
  line L88 (33.3, 19.05) -> (33.3, 18.4)
  line L89 (33.3, 19.05) -> (26.59, 19.05)
  line L90 (26.59, 19.05) -> (26.59, 22.75)
  line L91 (26.59, 22.75) -> (33.3, 22.75)
  line L92 (33.3, 22.75) -> (33.3, 19.05)
  line L93 (33.3, 22.75) -> (26.59, 22.75)
  line L94 (26.59, 22.75) -> (26.59, 23.4)
  line L95 (26.59, 23.4) -> (33.3, 23.4)
  line L96 (33.3, 23.4) -> (33.3, 22.75)
  line L97 (33.3, 23.4) -> (26.59, 23.4)
  line L98 (26.59, 23.4) -> (26.59, 24.45)
  line L99 (26.59, 24.45) -> (33.3, 24.45)
  line L100 (33.3, 24.45) -> (33.3, 23.4)
  point P0 (0, 0)
  dimension "d184" = 6.71
  dimension "d185" = 0.65
  dimension "d186" = 6.71
  dimension "d187" = 3.7
  dimension "d188" = 6.71
  dimension "d189" = 0.65
  dimension "d190" = 6.71
  dimension "d191" = 3.7
  dimension "d192" = 6.71
  dimension "d193" = 0.65
  dimension "d194" = 6.71
  dimension "d195" = 3.7
  dimension "d196" = 6.71
  dimension "d197" = 0.65
  dimension "d198" = 6.71
  dimension "d199" = 3.7
  dimension "d200" = 6.71
  dimension "d201" = 0.65
  dimension "d202" = 6.71
  dimension "d203" = 3.7
  dimension "d204" = 6.71
  dimension "d205" = 0.65
  dimension "d206" = 6.71
  dimension "d207" = 3.7
  dimension "d208" = 6.71
  dimension "d209" = 0.65
  dimension "d210" = 6.71
  dimension "d211" = 3.7
  dimension "d212" = 6.71
  dimension "d213" = 0.65
  dimension "d214" = 6.71
  dimension "d215" = 3.7
  dimension "d216" = 6.71
  dimension "d217" = 0.65
  dimension "d218" = 6.71
  dimension "d219" = 3.7
  dimension "d220" = 6.71
  dimension "d221" = 0.65
  dimension "d222" = 6.71
  dimension "d223" = 0.65
  dimension "d224" = 6.71
  dimension "d225" = 3.7
  dimension "d226" = 6.71
  dimension "d227" = 0.65
  dimension "d228" = 6.71
  dimension "d229" = 3.7
  dimension "d230" = 6.71
  dimension "d231" = 0.65
  constraints: 200 end point, 50 parallel, 25 horizontal, 25 perpendicular, 1 other
  measures "d184" distance of L2.end L3.end
  measures "d185" distance of L1.end L2.end
  measures "d186" distance of L6.end L7.end
  measures "d187" distance of L5.end L6.end
  measures "d188" distance of L10.end L11.end
  measures "d189" distance of L9.end L10.end
  measures "d190" distance of L14.end L15.end
  measures "d191" distance of L13.end L14.end
  measures "d192" distance of L18.end L19.end
  measures "d193" distance of L17.end L18.end
  measures "d194" distance of L22.end L23.end
  measures "d195" distance of L21.end L22.end
  measures "d196" distance of L26.end L27.end
  measures "d197" distance of L25.end L26.end
  measures "d198" distance of L30.end L31.end
  measures "d199" distance of L29.end L30.end
  measures "d200" distance of L34.end L35.end
  measures "d201" distance of L33.end L34.end
  measures "d202" distance of L38.end L39.end
  measures "d203" distance of L37.end L38.end
  measures "d204" distance of L42.end L43.end
  measures "d205" distance of L41.end L42.end
  measures "d206" distance of L46.end L47.end
  measures "d207" distance of L45.end L46.end
  measures "d208" distance of L50.end L51.end
  measures "d209" distance of L49.end L50.end
  measures "d210" distance of L54.end L55.end
  measures "d211" distance of L53.end L54.end
  measures "d212" distance of L58.end L59.end
  measures "d213" distance of L57.end L58.end
  measures "d214" distance of L62.end L63.end
  measures "d215" distance of L61.end L62.end
  measures "d216" distance of L66.end L67.end
  measures "d217" distance of L65.end L66.end
  measures "d218" distance of L70.end L71.end
  measures "d219" distance of L69.end L70.end
  measures "d220" distance of L74.end L75.end
  measures "d221" distance of L73.end L74.end
  measures "d222" distance of L79.end L78.end
  measures "d223" distance of L78.end L77.end
  measures "d224" distance of L82.end L83.end
  measures "d225" distance of L81.end L82.end
  measures "d226" distance of L86.end L87.end
  measures "d227" distance of L85.end L86.end
  measures "d228" distance of L90.end L91.end
  measures "d229" distance of L89.end L90.end
  measures "d230" distance of L94.end L95.end
  measures "d231" distance of L93.end L94.end
extrude "Extrusion16" cut sketch "Sketch19" against normal blind 18 contours L3 L6 L7 L0 | L11 L14 L15 L0 | L19 L22 L23 L0 | L27 L30 L31 L0 | L35 L38 L39 L0 | L43 L46 L47 L0 | L51 L54 L55 L0 | L59 L62 L63 L0 | L67 L70 L71 L0 | L75 L82 L83 L0 | L87 L90 L91 L0
sketch "Sketch20" plane through (0, 30, 0) normal (0, 1, 0) x (1, 0, 0)
  point P0 (0, 0)
body "Solid1"
